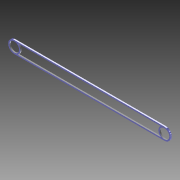
# Autodesk Inventor part: false chain
Saved by Autodesk Inventor 2011 (Build 150239000, 239)
## iProperties
Created: 2013-01-27
Part Number: false chain
Document SubType Name: Modeling
Designer: Danny
Density: 1 g/cm^3
Author: Danny
Autodesk Inventor part; units mm, degrees
ref_plane "YZ Plane" through (0, 0, 0) normal (1, 0, 0) x (0, 1, 0)
ref_plane "XZ Plane" through (0, 0, 0) normal (0, 1, 0) x (-1, 0, 0)
ref_plane "XY Plane" through (0, 0, 0) normal (0, 0, 1) x (1, 0, 0)
sketch "Sketch1" plane through (0, 0, 0) normal (0, 0, 1) x (1, 0, 0)
  circle A0 centre (0, 0) radius 18.8595
  arc A1 (0, 23.6903) -> (0, -23.6903) centre (0, 0) ccw
  circle A2 centre (584.2, 0) radius 18.8608
  arc A3 (569.8648, 18.8608) -> (569.8648, -18.8608) centre (584.2, 0) ccw
  line L0 (584.2, 23.6903) -> (0, 23.6903)
  line L1 (0, -23.6903) -> (584.2, -23.6903)
  line L2 (569.8648, -18.8608) -> (14.3352, -18.8608)
  line L3 (14.3352, 18.8608) -> (569.8648, 18.8608)
  arc A4 (14.3352, -18.8608) -> (14.3352, 18.8608) centre (0, 0) ccw
  arc A5 (584.2, -23.6903) -> (584.2, 23.6903) centre (584.2, 0) ccw
  dimension "d0" = 37.719
  constraints: 10 point on circle, 8 end point, 6 centre point, 6 tangent, 3 coincident, 2 parallel
  measures "d0" diameter of A0
extrude "Extrusion1" add sketch "Sketch1" along normal blind 5.08
body "Solid1"
